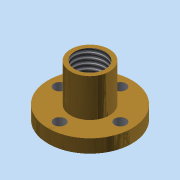
# Autodesk Inventor part: m8 nut
Saved by Autodesk Inventor 2015 (Build 190159000, 159)
## iProperties
Created: 2016-09-08
Part Number: m8 nut
Material: Generic
Document SubType Name: Modeling
Designer: Dustin
Density: 1 g/cm^3
Appearance: Default
Author: Dustin
Autodesk Inventor part; units mm, degrees
ref_plane "YZ Plane" through (0, 0, 0) normal (1, 0, 0) x (0, 1, 0)
ref_plane "XZ Plane" through (0, 0, 0) normal (0, 1, 0) x (-1, 0, 0)
ref_plane "XY Plane" through (0, 0, 0) normal (0, 0, 1) x (1, 0, 0)
sketch "Sketch1" plane through (0, 0, 0) normal (0, 0, 1) x (1, 0, 0)
  circle A0 centre (0, 0) radius 11
  dimension "d0" = 22
  constraints: 1 centre point, 1 coincident
  measures "d0" diameter of A0
extrude "Extrusion1" add sketch "Sketch1" along normal blind 3.5
sketch "Sketch2" plane through (0, 0, 3.5) normal (0, 0, 1) x (1, 0, 0)
  circle A0 centre (0, 0) radius 5.1
  dimension "d3" = 10.2
  constraints: 1 centre point, 1 coincident
  measures "d3" diameter of A0
extrude "Extrusion2" add sketch "Sketch2" along normal blind 10
sketch "Sketch3" plane through (0, 0, 3.5) normal (0, 0, 1) x (1, 0, 0)
  circle A0 centre (0, 0) radius 5.1 projected
  point P0 (0, 8)
  dimension "d7" = 8
  measures "d7" distance of point (0, 8) A0.centre
hole "Hole1" at (0, 8, 3.5) direction (0, 0, -1) diameter 3 depth 8 tip angle 118
pattern_circular "Circular Pattern1" count 4 over 360 about axis through (0, 0, 3.5) along (0, 0, 1) of "Hole1"
sketch "Sketch4" plane through (0, 0, 13.5) normal (0, 0, 1) x (1, 0, 0)
  circle A0 centre (0, 0) radius 4
  dimension "d18" = 8
  constraints: 1 centre point, 1 coincident
  measures "d18" diameter of A0
extrude "Extrusion3" cut sketch "Sketch4" against normal through all
thread "Thread1" size "M8x1.25" class "6H" standard "ANSI Metric M Profile" full length
body "Solid1"
